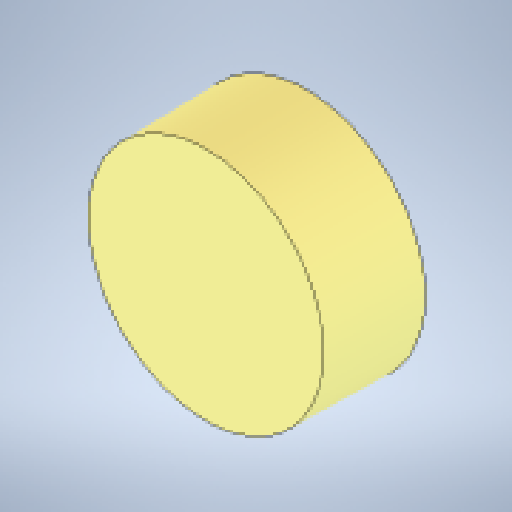
# Autodesk Inventor part: stopfen-front
Saved by Autodesk Inventor 2026.1 (Build 301233000, 233)
## iProperties
Created: 2019-03-04
Part Number: stopfen-front
Material: yellow foam
Document SubType Name: Modeling
Designer: rainer
Density: 1 g/cm^3
Appearance: Generic
Mass: 113.483 g
Surface Area: 141.81 cm^2
Volume: 113.483 cm^3
Author: rainer
Autodesk Inventor part; units mm, degrees
ref_plane "YZ Plane" through (0, 0, 0) normal (1, 0, 0) x (0, 1, 0)
ref_plane "XZ Plane" through (0, 0, 0) normal (0, 1, 0) x (-1, 0, 0)
ref_plane "XY Plane" through (0, 0, 0) normal (0, 0, 1) x (1, 0, 0)
sketch "Sketch1" plane through (0, 0, 0) normal (0, 0, 1) x (1, 0, 0)
  circle A0 centre (0, 0) radius 35.25
  circle A1 centre (0, 0) radius 40
  dimension "d0" = 70.5
  dimension "d4" = 80
  constraints: 2 centre point, 2 coincident
  measures "d0" diameter of A0
  measures "d4" diameter of A1
extrude "Extrusion1" add sketch "Sketch1" along normal blind 29.5 contours A0
draft "FaceDraft1" angle 1 pull direction (0, 0, 1) faces at (35.144, -2.7316, 19.6667) fixed edges at (-35.25, 0, 0)
extrude "Extrusion2" add sketch "Sketch1" along normal mid plane 20 contours A0 | A1
sketch "Skizze2" plane through (0, 0, 29.5) normal (0, 0, 1) x (1, 0, 0)
  circle A0 centre (0, 0) radius 34.7351 projected
  line L0 (-21.0374, 27.6397) -> (-15.0374, 27.6397)
  line L1 (-15.0374, 27.6397) -> (-15.0374, 26.6397)
  line L2 (-15.0374, 26.6397) -> (-21.0374, 26.6397)
  line L3 (-21.0374, 26.6397) -> (-21.0374, 27.6397)
  line L4 (-15.0374, 26.6397) -> (14.9626, 26.6397)
  line L5 (14.9626, 26.6397) -> (14.9626, -29.8603)
  line L6 (14.9626, -29.8603) -> (-15.0374, -29.8603)
  line L7 (-15.0374, -29.8603) -> (-15.0374, 26.6397)
  line L8 (-15.0374, 26.6397) -> (14.9626, 26.6397)
  line L9 (14.9626, 26.6397) -> (14.9626, 29.6397)
  line L10 (14.9626, 29.6397) -> (-15.0374, 29.6397)
  line L11 (-15.0374, 29.6397) -> (-15.0374, 26.6397)
  dimension "d7" = 6
  dimension "d8" = 1
  dimension "d9" = 30
  dimension "d10" = 56.5
  dimension "d11" = 3
  constraints: 24 end point, 6 parallel, 3 horizontal, 3 perpendicular, 2 other
  measures "d7" distance of L1.end L2.end
  measures "d8" distance of L0.end L1.end
  measures "d9" distance of L5.end L6.end
  measures "d10" distance of L4.end L5.end
  measures "d11" distance of L9.end L8.end
extrude "Extrusion3" cut sketch "Skizze2" against normal blind 15 contours L11 L10 L9 L4 L1 | L4 L5 L6 L7
body "Solid1"
